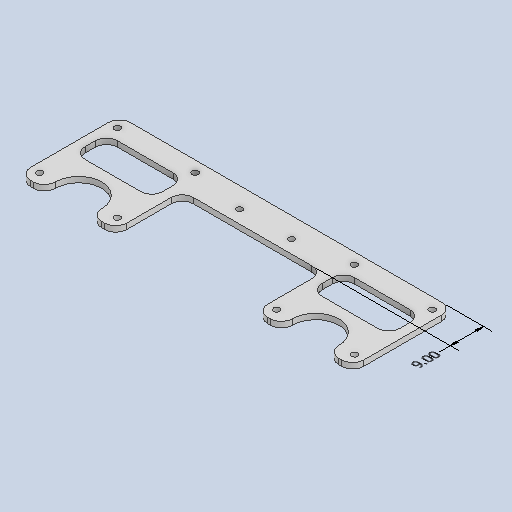
# Autodesk Inventor part: hipjoint_upper
Saved by Autodesk Inventor 2024.1 (Build 281209000, 209)
## iProperties
Created: 2024-10-08
Part Number: hipjoint_upper
Material: 一般
Document SubType Name: Sheet Metal
Designer: hibik
Density: 1 g/cm^3
Sheet Metal Rule: Default_mm
Appearance: 既定
Author: hibik
Autodesk Inventor part; units mm, degrees
ref_plane "YZ Plane" through (0, 0, 0) normal (1, 0, 0) x (0, 1, 0)
ref_plane "XZ Plane" through (0, 0, 0) normal (0, 1, 0) x (-1, 0, 0)
ref_plane "XY Plane" through (0, 0, 0) normal (0, 0, 1) x (1, 0, 0)
sketch "スケッチ2" plane through (0, 0, 0) normal (0, 1, 0) x (-1, 0, 0)
  line L0 (19, 24) -> (45, 24)
  line L1 (45, 24) -> (45, 0)
  line L2 (45, 0) -> (19, 0)
  line L3 (19, 0) -> (19, 24)
  circle A0 centre (32, 24) radius 6.25
  line L4 (19, 24) -> (45, 24)
  line L5 (45, 24) -> (45, 27)
  line L6 (45, 27) -> (19, 27)
  line L7 (19, 27) -> (19, 24)
  line L8 (-45, 24) -> (-19, 24)
  line L9 (-19, 24) -> (-19, 0)
  line L10 (-19, 0) -> (-45, 0)
  line L11 (-45, 0) -> (-45, 24)
  circle A1 centre (-32, 24) radius 6.25
  line L12 (-45, 24) -> (-19, 24)
  line L13 (-19, 24) -> (-19, 27)
  line L14 (-19, 27) -> (-45, 27)
  line L15 (-45, 27) -> (-45, 24)
  line L16 (0, -6.05) -> (0, 36.3)
  line L17 (64.3086, 0) -> (-70.8513, 0)
  line L18 (-19, 9) -> (19, 9)
  line L19 (19, 9) -> (19, 0)
  line L20 (19, 0) -> (-19, 0)
  line L21 (-19, 0) -> (-19, 9)
  point P0 (0, 0)
  point P1 (-51.5428, 0.5174)
  point P2 (19, 0)
  point P3 (37.4829, 27)
  point P4 (26.5171, 27)
  point P5 (-26.5171, 27)
  point P6 (-37.4829, 27)
  point P7 (-19, 0)
  dimension "d4" = 26
  dimension "d5" = 24
  dimension "d6" = 12.5
  dimension "d7" = 3
  dimension "d8" = 26
  dimension "d9" = 24
  dimension "d10" = 12.5
  dimension "d11" = 3
  dimension "d12" = 64
  dimension "d13" = 9
  measures "d4" distance of L1.end L2.end
  measures "d5" distance of L0.end L1.end
  measures "d6" diameter of A0
  measures "d7" distance of L4.end L5.end
  measures "d8" distance of L9.end L10.end
  measures "d9" distance of L8.end L9.end
  measures "d10" diameter of A1
  measures "d11" distance of L12.end L13.end
  measures "d12" distance of A0.centre point (-32, 24)
  measures "d13" distance between parallel lines of L17 L18
extrude "プレート2" add sketch "スケッチ2" along normal blind 1.5 contours A0 L6 L5 L0 | L0 L1 L2 L3 A0 | L0 L7 L6 A0 | L17 L16 L18 L3 | L17 L9 L18 L16 | L10 L11 L8 A1 L9 | L8 A1 L14 L13 | L15 L14 A1 L8
sketch "スケッチ3" plane through (0, 1.5, 0) normal (0, 1, 0) x (1, 0, 0)
  line L0 (45, 0) -> (45, -27) projected
  line L1 (19, -27) -> (19, -9) projected
  line L2 (-42.5, -3) -> (-21.5, -3)
  line L3 (-21.5, -3) -> (-21.5, -17.75)
  line L4 (-21.5, -17.75) -> (-42.5, -17.75)
  line L5 (-42.5, -17.75) -> (-42.5, -3)
  line L6 (21.5, -3) -> (42.5, -3)
  line L7 (42.5, -3) -> (42.5, -17.75)
  line L8 (42.5, -17.75) -> (21.5, -17.75)
  line L9 (21.5, -17.75) -> (21.5, -3)
  arc A0 (-26.5171, -27) -> (-37.4829, -27) centre (-32, -24) ccw projected
  line L10 (-42.5, -6) -> (-21.5, -6)
  line L11 (-21.5, -6) -> (-21.5, -14.75)
  line L12 (-21.5, -14.75) -> (-42.5, -14.75)
  line L13 (-42.5, -14.75) -> (-42.5, -6)
  line L14 (21.5, -6) -> (42.5, -6)
  line L15 (42.5, -6) -> (42.5, -14.75)
  line L16 (42.5, -14.75) -> (21.5, -14.75)
  line L17 (21.5, -14.75) -> (21.5, -6)
  circle A1 centre (-42.5, -24) radius 0.85 projected
  circle A2 centre (-42.5, -3) radius 0.85 projected
  circle A3 centre (-21.5, -3) radius 0.85 projected
  circle A4 centre (-21.5, -24) radius 0.85 projected
  circle A5 centre (21.5, -24) radius 0.85 projected
  circle A6 centre (42.5, -24) radius 0.85 projected
  circle A7 centre (42.5, -3) radius 0.85 projected
  circle A8 centre (21.5, -3) radius 0.85 projected
  circle A9 centre (7, -5.5) radius 0.8 projected
  circle A10 centre (-7, -5.5) radius 0.8 projected
  arc A11 (37.4829, -27) -> (26.5171, -27) centre (32, -24) ccw projected
  arc A12 (37.4829, -27) -> (26.5171, -27) centre (32, -24) ccw projected
  line L18 (45, -27) -> (37.4829, -27) projected
  line L19 (-45, 0) -> (45, 0) projected
  line L20 (-45, -27) -> (-45, 0) projected
  line L21 (-37.4829, -27) -> (-45, -27) projected
  arc A13 (-26.5171, -27) -> (-37.4829, -27) centre (-32, -24) ccw projected
  line L22 (-19, -27) -> (-26.5171, -27) projected
  line L23 (-19, -9) -> (-19, -27) projected
  line L24 (19, -9) -> (-19, -9) projected
  line L25 (26.5171, -27) -> (19, -27) projected
  point P0 (0, 0)
  dimension "d20" = 3
  dimension "d21" = 3
  constraints: 32 end point, 8 parallel, 6 point on line, 4 coincident, 4 horizontal, 4 perpendicular, 2 tangent
  measures "d20" distance between parallel lines of L6 L14
  measures "d21" distance between parallel lines of L8 L16
extrude "切り取り1" cut sketch "スケッチ3" against normal blind 1.5 contours L16 L9 L14 L7 | L12 L5 L10 L3 | A7 L6 L7 | L7 L6 A7 | A8 L6 L9 | L9 L6 A8 | A3 L2 L3 | L3 L2 A3 | A2 L2 L5 | L5 L2 A2 | A1 | A4 | A5 | A6 | A9 | A10
fillet "フィレット1" radius 3 20 edges at (-21.5, 0.75, 6) (-21.5, 0.75, 14.75) (-42.5, 0.75, 14.75) (-42.5, 0.75, 6) (-37.4829, 0.75, 27) (-45, 0.75, 27) (-26.5171, 0.75, 27) (-19, 0.75, 27) (19, 0.75, 27) (26.5171, 0.75, 27) (37.4829, 0.75, 27) (45, 0.75, 27) (45, 0.75, 0) (-45, 0.75, 0) (-19, 0.75, 9) (19, 0.75, 9) (42.5, 0.75, 14.75) (21.5, 0.75, 14.75) (21.5, 0.75, 6) (42.5, 0.75, 6)
equation "\"d11\" = d7"
equation "\"d18\" = Thickness"
equation "\"d14\" = Thickness"
equation "\"BendRadius\" = Thickness"
equation "\"BendReliefWidth\" = Thickness"
equation "\"BendReliefDepth\" = 0.5 * Thickness"
equation "\"CornerReliefSize\" = 4 * Thickness"
equation "\"MinimumRemnant\" = 2 * Thickness"
equation "\"TransitionRadius\" = BendRadius"
equation "\"JacobiRadiusSize\" = BendRadius"
equation "\"GapSize\" = Thickness"
equation "\"Thickness\" = 1.5"
